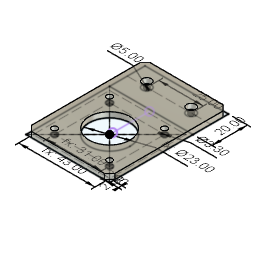
stepper mount with parameter v1 (Autodesk Fusion 360 design; units mm, degrees)
Autodesk Fusion 360 part; units mm, degrees
sketch "Skizze1" plane through (0, 0, 0) normal (0, 0, 1) x (1, 0, 0)
  circle A0 centre (0, 0) radius 11.5
  line L0 (23.5, -23.5) -> (-23.5, -23.5)
  line L1 (-23.5, -23.5) -> (-23.5, 23.5)
  line L2 (-23.5, 23.5) -> (23.5, 23.5)
  line L3 (23.5, 23.5) -> (23.5, -23.5)
  line L4 (23.5, -23.5) -> (-23.5, 23.5) construction
  line L5 (-23.5, -23.5) -> (23.5, 23.5) construction
  line L6 (21.5, -21.5) -> (-21.5, -21.5) construction
  line L7 (-21.5, -21.5) -> (-21.5, 21.5) construction
  line L8 (-21.5, 21.5) -> (21.5, 21.5) construction
  line L9 (21.5, 21.5) -> (21.5, -21.5) construction
  line L10 (21.5, -21.5) -> (-21.5, 21.5) construction
  line L11 (-21.5, -21.5) -> (21.5, 21.5) construction
  line L12 (15.5, -15.5) -> (-15.5, -15.5) construction
  line L13 (-15.5, -15.5) -> (-15.5, 15.5) construction
  line L14 (-15.5, 15.5) -> (15.5, 15.5) construction
  line L15 (15.5, 15.5) -> (15.5, -15.5) construction
  line L16 (15.5, -15.5) -> (-15.5, 15.5) construction
  line L17 (-15.5, -15.5) -> (15.5, 15.5) construction
  circle A1 centre (-15.5, 15.5) radius 1.65
  circle A2 centre (15.5, 15.5) radius 1.65
  circle A3 centre (15.5, -15.5) radius 1.65
  circle A4 centre (-15.5, -15.5) radius 1.65
  line L18 (-23.5, 23.5) -> (-23.5, 43.5)
  line L19 (-23.5, 43.5) -> (23.5, 43.5)
  line L20 (23.5, 43.5) -> (23.5, 23.5)
  line L21 (-23.5, 33.5) -> (23.5, 33.5) construction
  circle A5 centre (-12.5, 33.5) radius 2.5
  circle A6 centre (12.5, 33.5) radius 2.5
  line L22 (0, 1.75) -> (0, 22.5)
  dimension "d120" = 43
  dimension "d121" = 23
  dimension "d122" = 2
  dimension "d123" = 31
  dimension "d124" = 3.3
  dimension "d125" = 2
  dimension "d126" = 20
  dimension "d127" = 5
  dimension "d128" = 25
  constraint coincident A0.centre origin
  constraint horizontal L0
  constraint perpendicular L0 L1
  constraint parallel L0 L2
  constraint parallel L1 L3
  constraint coincident L4 A0.centre
  constraint coincident L5 A0.centre
  constraint horizontal L6
  constraint perpendicular L6 L7
  constraint parallel L6 L8
  constraint parallel L7 L9
  constraint coincident L10 A0.centre
  constraint coincident L11 A0.centre
  constraint equal L6 L9
  constraint horizontal L12
  constraint perpendicular L12 L13
  constraint parallel L12 L14
  constraint parallel L13 L15
  constraint coincident L16 A0.centre
  constraint coincident L17 A0.centre
  constraint equal L12 L15
  constraint coincident L13.end L14.start
  constraint coincident L14.end L15.start
  constraint coincident L12.start L15.end
  constraint coincident L12.end L13.start
  constraint equal A1 A4
  constraint equal A3 A4
  constraint equal A2 A3
  constraint perpendicular L2 L18
  constraint perpendicular L3 L19
  constraint vertical L20
  constraint midpoint L18 L21.start
  constraint midpoint L20 L21.end
  constraint coincident L21 A5.centre
  constraint coincident L21 A6.centre
  constraint equal A5 A6
  constraint symmetric A5 A6 L22
  measures "d120" distance of L6.start L6.end
  measures "d121" diameter of A0
  measures "d122" horizontal distance of L0.start L6.start
  measures "d123" distance of L12.start L12.end
  measures "d124" diameter of A2
  measures "d125" vertical distance of L0.start L6.start
  measures "d126" distance of L2.end L19.end
  measures "d127" diameter of A5
  measures "d128" distance of A5.centre A6.centre
extrude "Extrusion1" add sketch "Skizze1" along normal blind 3
chamfer "Fase1" distance 3 angle 45 4 edges at (-23.5, -23.5, 1.5) (23.5, -23.5, 1.5) (23.5, 43.5, 1.5) (-23.5, 43.5, 1.5)
equation "_content = 1" comment "ultimate fusion 360 parameter table for 3d printer"
equation "_author = 1" comment "Thomas Dragon"
equation "_version = 1" comment "V 1.0 2021-03-13"
equation "_outer_dimensions = 1" comment "--- placeholder delimiter ---"
equation "frame_outer_x = 400 mm" comment "external dimensions"
equation "frame_outer_y = 400 mm" comment "external dimensions"
equation "frame_outer_z = 600 mm" comment "external dimensions"
equation "_threaded_screws = 1" comment "--- placeholder delimiter ---"
equation "M3_hole_dia = 3.5 mm" comment "for printing parts"
equation "M4_hole_dia = 4.5 mm" comment "for printing parts"
equation "M5_hole_dia = 5.2 mm" comment "for printing parts"
equation "M6_hole_dia = 6.2 mm" comment "for printing parts"
equation "M3_hole_dia_thread = 2.6 mm" comment "for printing parts to screw"
equation "M4_hole_dia_thread = 3.4 mm" comment "for printing parts to screw"
equation "M5_hole_dia_thread = 4.3 mm" comment "for printing parts to screw"
equation "M6_hole_dia_thread = 5.2 mm" comment "for printing parts to screw"
equation "M3_head_dia = 6 mm" comment "for printing parts"
equation "M4_head_dia = 7 mm" comment "for printing parts"
equation "M5_head_dia = 9 mm" comment "for printing parts"
equation "M6_head_dia = 11 mm" comment "for printing parts"
equation "M3_head_height = 3 mm" comment "for printing parts"
equation "M4_head_height = 4 mm" comment "for printing parts"
equation "M5_head_height = 5 mm" comment "for printing parts"
equation "M6_head_height = 6 mm" comment "for printing parts"
equation "_stepper = 1" comment "--- placeholder delimiter ---"
equation "nema_17_outer_XY = 43 mm" comment "nema 17 stepper"
equation "nema_17_outer_z = 40 mm" comment "nema 17 stepper"
equation "nema_17_screw_distance = 31 mm" comment "nema 17 stepper"
equation "nema_17_center_ring_dia = 23 mm" comment "nema 17 stepper"
equation "nema_17_center_ring_height = 2 mm" comment "nema 17 stepper"
equation "nema_17_shaft_length = 24 mm" comment "nema 17 stepper"
equation "nema_17_shaft_dia = 5 mm" comment "nema 17 stepper"
equation "_bearing = 1" comment "--- placeholder delimiter ---"
equation "lm8uu_outer_dia = 15 mm" comment "bearing lm8uu"
equation "lm8uu_length = 24 mm" comment "bearing lm8uu"
equation "lm8uu_nut_distance_cc = 16.4 mm" comment "bearing lm8uu"
equation "scs8uu_lenght = 30 mm" comment "bearing scs8uu"
equation "scs8uu_width = 34.4 mm" comment "bearing scs8uu"
equation "scs8uu_screw_distance_cc_1 = 18 mm" comment "bearing scs8uu parallel to the rod"
equation "scs8uu_screw_distance_cc_2 = 24 mm" comment "bearing scs8uu perpendicular to the rod"
equation "scs8uu_base_road_cc = 11 mm" comment "bearing scs8uu distance base to center rod"
equation "scs8uu_screw_hole_dia = 4 mm" comment "M4 mounting"
equation "lmk8luu_length = 45 mm" comment "long flange bearing"
equation "lmk8luu_head_xy = 25 mm" comment "long flange bearing"
equation "lmk8luu_body_dia = 15 mm" comment "long flange bearing"
equation "lmk8luu_circle_holes_dia = 24 mm" comment "long flange bearing"
equation "lmk8luu_screw_hole_dia = 3 mm" comment "M3 mounting"
equation "_mounting = 1" comment "--- placeholder delimiter ---"
equation "kp08_screw_distance_cc = 42 mm" comment "pillow block bearing"
equation "kp08_base_road_cc = 15 mm" comment "distance base to center rod"
equation "kp08_screw_hole_dia = 4 mm" comment "M4 mounting"
equation "sk8_screw_distance_cc = 32 mm" comment "end support for shaft"
equation "sk8_base_road_cc = 20 mm" comment "distance base to center rod"
equation "sk8_screw_hole_dia = 5 mm" comment "M5 mounting"
equation "_trapezoidal_screw = 1" comment "--- placeholder delimiter ---"
equation "trapezoidal_screw_z_length = 300 mm" comment "trapezoidal_screw"
equation "coupler_5x8_length = 25 mm" comment "5x8 coupler"
equation "coupler_5x8_outer_dia = 19 mm" comment "5x8 coupler"
equation "t8_nut_outer_dia_1 = 22 mm" comment "T8 Lead Screw Nut"
equation "t8_nut_outer_dia_2 = 10.2 mm" comment "T8 Lead Screw Nut"
equation "t8_nut_screw_hole_dia = 3 mm" comment "M3 mounting"
equation "t8_nut_screw_circle_holes_dia = 16 mm" comment "with 4 screw holes"
equation "_headbed = 1" comment "--- placeholder delimiter ---"
equation "heatbed_outer_x = 220 mm" comment "heatbed"
equation "heatbed_outer_y = 220 mm" comment "heatbed"
equation "heatbed_x_srew_cc = 210 mm" comment "heatbed"
equation "heatbed_y_srew_cc = 210 mm" comment "heatbed"
equation "_steal_rods = 1" comment "--- placeholder delimiter ---"
equation "x_rods_distance_cc = 40 mm"
equation "y_rods_distance_cc = 140 mm"
equation "z_rods_distance_cc = 300 mm"
equation "steel_rods_dia = 8.2 mm" comment "for printing parts"
equation "_profiles = 1" comment "--- placeholder delimiter ---"
equation "x_profile_distance_cc = 60 mm" comment "alu extrusion profile"
equation "y_profile_distance_cc = 160 mm" comment "alu extrusion profile"
equation "z_profile_distance_cc = 300 mm" comment "alu extrusion profile"
equation "x_profile_length = 300 mm" comment "alu extrusion profile"
equation "y_profile_length = 300 mm" comment "alu extrusion profile"
equation "z_profile_length = 300 mm" comment "alu extrusion profile"
equation "y_profile_xy = 20 mm" comment "alu extrusion profile"
equation "z_profil_x = 20 mm" comment "alu extrusion profile"
equation "z_profil_y = 40 mm" comment "alu extrusion profile"
equation "profil_nut_width = 6 mm" comment "for t nut 6mm 20mm profil"
equation "profil_nut_depth = 5 mm" comment "fot t nut 6mm 20mm profil"
equation "_pulley = 1" comment "--- placeholder delimiter ---"
equation "pulley_gt2_20t_outer_dia = 16 mm" comment "20 teeth m4 mounting"
equation "pulley_gt2_20t_inner_dia = 12.2 mm" comment "20 teeth m4 mounting"
equation "pulley_gt2_16t_outer_dia = 13.8 mm" comment "16 teeth m3 mounting"
equation "pulley_gt2_16t_inner_dia = 9.4 mm" comment "16 teeth m3 mounting"
equation "_e3d_hot_end_175 = 1" comment "--- placeholder delimiter ---"
equation "e3d_heigh_all = 62.3 mm" comment "e3d"
equation "e3d_mounting_dia_inner = 12 mm" comment "e3d"
equation "e3d_mounting_dia_outer = 16 mm" comment "e3d"
equation "e3d_mounting_height = 6 mm" comment "e3d"
equation "e3d_upper_mount_height = 3.7 mm" comment "e3d"
equation "e3d_distance_nozzle_mounting_center = e3d_heigh_all - ( e3d_mounting_height / 2 ) - e3d_upper_mount_height" comment "= distance headbed to nozzle"
equation "_flanged_ball_bearing = 1" comment "--- placeholder delimiter ---"
equation "f624_zz_outer_dia = 15 mm" comment "4x13x5 mm suitable for gt2 pulley 20"
equation "f624_zz_inner_dia = 13 mm" comment "4x13x5 mm suitable for gt2 pulley 20"
equation "f624_zz_hole_dia = 4 mm" comment "M4 mounting"
equation "f623_zz_outer_dia = 11.5 mm" comment "3x10x4 mm suitable for gt2 pulley 16"
equation "f623_zz_inner_dia = 10 mm" comment "3x10x4 mm suitable for gt2 pulley 16"
equation "f623_zz_hole_dia = 3 mm" comment "M3 mounting"
equation "_standard_fans = 1" comment "--- placeholder delimiter ---"
equation "fan_30x30_xy_outside = 30 mm" comment "30x30 standard fan m3 mounting"
equation "fan_30x30_xy_screw_distance = 24 mm" comment "30x30 standard fan"
equation "fan_30x30_fan_opening_dia = 28 mm" comment "30x30 standard fan"
equation "fan_40x40_xy_outside = 40 mm" comment "40x40 standard fan m3 mounting"
equation "fan_40x40_xy_screw_distance = 32 mm" comment "40x40 standard fan"
equation "fan_40x40_fan_opening_dia = 38 mm" comment "40x40 standard fan"
equation "fan_50x50_xy_outside = 50 mm" comment "50x50 standard fan m3 mounting"
equation "fan_50x50_xy_screw_distance = 40 mm" comment "50x50 standard fan"
equation "fan_50x50_fan_opening_dia = 47 mm" comment "60x60 standard fan"
equation "fan_60x60_xy_outside = 60 mm" comment "60x60 standard fan m4 mounting"
equation "fan_60x60_xy_screw_distance = 51 mm" comment "60x60 standard fan"
equation "fan_60x60_fan_opening_dia = 57 mm" comment "60x60 standard fan"
equation "fan_12x120_xy_outside = 120 mm" comment "12x120 standard fan m4 mounting"
equation "fan_12x120_xy_screw_distance = 105 mm" comment "12x120 standard fan"
equation "fan_12x120_fan_opening_dia = 116 mm" comment "12x120 standard fan"
equation "d120 = nema_17_outer_XY"
equation "d121 = nema_17_center_ring_dia"
equation "d123 = nema_17_screw_distance"
